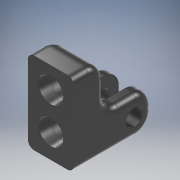
# Autodesk Inventor part: Y-Axis_Belt_Bearing_Mount_LM3045
Saved by Autodesk Inventor 2020.3 (Build 243373000, 373)
## iProperties
Created: 2020-05-31
Part Number: Y-Axis_Belt_Bearing_Mount_LM3045
Material: ABS Plastic
Document SubType Name: Modeling
Designer: rah75
Density: 1.06 g/cm^3
Appearance: Satin - Black
Author: rah75
Autodesk Inventor part; units mm, degrees
ref_plane "YZ Plane" through (0, 0, 0) normal (1, 0, 0) x (0, 1, 0)
ref_plane "XZ Plane" through (0, 0, 0) normal (0, 1, 0) x (-1, 0, 0)
ref_plane "XY Plane" through (0, 0, 0) normal (0, 0, 1) x (1, 0, 0)
sketch "Sketch1" plane through (0, 0, 0) normal (1, 0, 0) x (0, 1, 0)
  line L0 (-13.5, 12.925) -> (13.5, 12.925)
  line L1 (13.5, 12.925) -> (13.5, -12.925)
  line L2 (13.5, -12.925) -> (-13.5, -12.925)
  line L3 (-13.5, -12.925) -> (-13.5, 12.925)
  line L4 (-13.5, 12.925) -> (13.5, -12.925) construction
  line L5 (13.5, 12.925) -> (-13.5, -12.925) construction
  circle A0 centre (-7.65, -7.075) radius 8 construction
  line L6 (-5.5, 12.925) -> (-5.5, 10.887)
  circle A1 centre (-7.65, -7.075) radius 2.75
  line L7 (-1.8, -12.925) -> (-1.8, -2.075)
  arc A2 (3.2, 2.925) -> (-1.8, -2.075) centre (3.2, -2.075) ccw
  line L8 (3.2, 2.925) -> (13.5, 2.925)
  point P0 (0, 0)
  dimension "d0" = 27
  dimension "d1" = 25.85
  dimension "d2" = 16
  dimension "d3" = 21.15
  dimension "d4" = 19
  dimension "d5" = 20
  dimension "d6" = 5.5
  dimension "d7" = 5.85
  dimension "d8" = 5.85
  dimension "d9" = 5.85
  dimension "d10" = 10
  dimension "d11" = 5
  constraints: 18 end point, 3 centre point, 3 point on line, 2 midpoint, 2 parallel, 2 perpendicular, 2 point on circle, 2 tangent, 2 vertical, 1 coincident, 1 horizontal
  measures "d0" distance of L1.end L2.end
  measures "d1" distance of L0.end L1.end
  measures "d2" diameter of A0
  measures "d3" distance from line of A0.centre L1
  measures "d4" distance between parallel lines of L6 L1
  measures "d5" distance from line of A0.centre L0
  measures "d6" diameter of A1
  measures "d7" distance from line of L3 A0.centre
  measures "d8" distance from line of L2 A0.centre
  measures "d9" distance from line of L7 A0.centre
  measures "d10" distance between parallel lines of L0 L8
  measures "d11" radius of A2
extrude "Extrusion1" add sketch "Sketch1" along normal mid plane 15 contours L0 L1 L8 A2 L7 L2 L3
fillet "Fillet1" radius 5 3 edges at (0, -1.8, -12.925) (0, -13.5, -12.925) (0, 13.5, 2.925)
sketch "Sketch2" plane through (0, 0, 0) normal (1, 0, 0) x (0, 1, 0)
  arc A0 (8.5, 2.925) -> (13.5, 7.925) centre (8.5, 7.925) ccw projected
  line L0 (13.5, 7.925) -> (13.5, 12.925) projected
  line L1 (13.5, 12.925) -> (-13.5, 12.925) projected
  line L2 (-13.5, 12.925) -> (-13.5, -7.925) projected
  arc A1 (-13.5, -7.925) -> (-8.5, -12.925) centre (-8.5, -7.925) ccw projected
  line L3 (-8.5, -12.925) -> (-6.8, -12.925) projected
  arc A2 (-6.8, -12.925) -> (-1.8, -7.925) centre (-6.8, -7.925) ccw projected
  line L4 (-1.8, -7.925) -> (-1.8, -2.075) projected
  arc A3 (3.2, 2.925) -> (-1.8, -2.075) centre (3.2, -2.075) ccw projected
  line L5 (3.2, 2.925) -> (8.5, 2.925) projected
  circle A4 centre (-7.65, -7.075) radius 2.75 projected
  circle A5 centre (-7.65, -7.075) radius 10
  point P0 (0, 0)
  dimension "d15" = 20
  constraints: 1 centre point, 1 coincident
  measures "d15" diameter of A5
extrude "Extrusion2" cut sketch "Sketch2" against normal mid plane 7 contours A5 L2 A1 L3 A2 L4 A3 | A3 L4 A2 L3 A1 L2 A5 | A4
fillet "Fillet2" radius 5 2 edges at (0, -1.0981, 0.4797) (0, -13.5, 1.0353)
sketch "Sketch3" plane through (-7.5, -13.5, 12.925) normal (0, 0, 1) x (1, 0, 0)
  line L0 (0, 27) -> (15, 27) projected
  point P0 (7.5, 13.5)
  point P1 (7.5, 20)
  point P2 (7.5, 8)
  dimension "d19" = 7
  dimension "d20" = 19
  constraints: 2 vertical alignment
  measures "d19" distance from line of point (7.5, 20) L0
  measures "d20" distance from line of point (7.5, 8) L0
hole "Hole1" at (0, 6.5, 12.925) at (0, -5.5, 12.925) direction (0, 0, -1) diameter 7.8 depth 6.7 countersink diameter 8.3 countersink angle 8
sketch "Sketch4" plane through (-7.5, -13.5, 12.925) normal (0, 0, 1) x (1, 0, 0)
  circle A0 centre (7.5, 20) radius 3.9 projected
  circle A1 centre (7.5, 8) radius 3.9 projected
  point P0 (7.5, 13.5)
  constraints: 2 coincident
hole "Hole2" at (0, 6.5, 12.925) at (0, -5.5, 12.925) direction (0, 0, -1) diameter 5.5 end through all clearance for "Flat Head Machine Screw" size "M5" standard "Ansi Metric M Profile"
fillet "Fillet3" radius 2 18 edges at (7.5, 5.85, 2.925) (7.5, -0.3355, 1.4605) (7.5, -1.8, -5) (7.5, -3.2645, -11.4605) (7.5, -7.65, -12.925) (7.5, -12.0355, -11.4605) (7.5, -13.5, 2.5) (7.5, 13.5, 10.425) (7.5, 12.0355, 4.3895) (-7.5, 13.5, 10.425) (-7.5, 5.85, 2.925) (-7.5, -0.3355, 1.4605) (-7.5, -1.8, -5) (-7.5, -3.2645, -11.4605) (-7.5, -7.65, -12.925) (-7.5, -12.0355, -11.4605) (-7.5, -13.5, 2.5) (-7.5, 12.0355, 4.3895)
equation "\"d8\" = d7"
equation "\"d9\" = d7"
body "Solid1"
